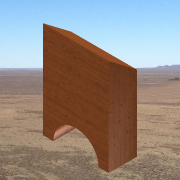
# Autodesk Inventor part: 2p4irsh
Saved by Autodesk Inventor 2013 SP2 (Build 170200200, 200)
## iProperties
Company: HERA Project
Created: 2013-12-04
Part Number: 2p4irsh
Material: Wood (Cherry)
Document SubType Name: Modeling
Designer: David DeBoer
Mass: 283.669 g
Surface Area: 501.887 cm^2
Volume: 567.338 cm^3
Density: 0.5 g/cm^3
Description: intermediate rim spar holder
Author: David DeBoer
Autodesk Inventor part; units mm, degrees
ref_plane "YZ Plane" through (0, 0, 0) normal (1, 0, 0) x (0, 1, 0)
ref_plane "XZ Plane" through (0, 0, 0) normal (0, 1, 0) x (-1, 0, 0)
ref_plane "XY Plane" through (0, 0, 0) normal (0, 0, 1) x (1, 0, 0)
sketch "Sketch1" plane through (0, 0, 0) normal (1, 0, 0) x (0, 1, 0)
  line L0 (0, 0) -> (131.191, 0)
  line L1 (0, 0) -> (0, -38.1)
  line L2 (0, -38.1) -> (102.2096, -38.1)
  line L3 (131.191, 0) -> (102.2096, -38.1)
  dimension "d2" = 131.191
  dimension "d4" = 38.1
  dimension "d5" = 102.2096
  constraints: 8 end point, 2 perpendicular, 1 horizontal
  measures "d2" distance of L0.start L0.end
  measures "d4" distance of L0.start L1.end
  measures "d5" distance of L1.end L2.end
extrude "Extrusion1" add sketch "Sketch1" along normal blind 88.9
sketch "Sketch2" plane through (0, 0, 0) normal (0, 0, 1) x (1, 0, 0)
  line L0 (0, 0) -> (88.9, 0) projected
  circle A0 centre (44.45, 0) radius 30.48
  dimension "d8" = 60.96
  constraints: 1 centre point, 1 midpoint
  measures "d8" diameter of A0
extrude "Extrusion2" cut sketch "Sketch2" against normal blind 88.9
sketch "Sketch3" plane through (0, 131.191, 0) normal (0, 0.7959065, -0.6054195) x (1, 0, 0)
  line L0 (0, 0) -> (88.9, 0) projected
  line L1 (88.9, 47.8699) -> (88.9, 0) projected
  circle A0 centre (63.5, 23.9406) radius 3.175
  circle A1 centre (25.4, 23.9406) radius 3.175
  point P0 (0, 79.4256)
  dimension "d11" = 25.4
  dimension "d14" = 38.1
  constraints: 2 centre point, 1 horizontal, 2 other
  measures "d11" distance from line of L1 A0.centre
  measures "d14" distance of A0.centre A1.centre
hole "Hole1" at (25.4, 116.6969, -19.0545) at (63.5, 116.6969, -19.0545) direction (0, -0.7959065, 0.6054195) diameter 3.175 depth 25.4 tip angle 118
body "Solid1"
